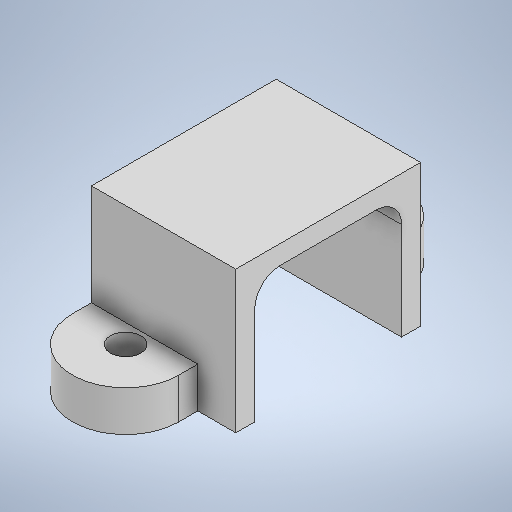
# Autodesk Inventor part: soporteMotor
Saved by Autodesk Inventor 2025.2 (Build 292293000, 293)
## iProperties
Created: 2025-06-11
Part Number: soporteMotor
Material: Generic
Document SubType Name: Modeling
Designer: cdavi
Density: 1 g/cm^3
Appearance: Default
Author: cdavi
Autodesk Inventor part; units mm, degrees
ref_plane "YZ Plane" through (0, 0, 0) normal (1, 0, 0) x (0, 1, 0)
ref_plane "XZ Plane" through (0, 0, 0) normal (0, 1, 0) x (-1, 0, 0)
ref_plane "XY Plane" through (0, 0, 0) normal (0, 0, 1) x (1, 0, 0)
sketch "Sketch1" plane through (0, 0, 0) normal (1, 0, 0) x (0, 1, 0)
  line L0 (11.2, 0) -> (11.2, -7.3)
  line L1 (11.2, -7.3) -> (0, -7.3)
  line L2 (9.7, 0) -> (9.7, -3.8)
  line L3 (7.7, -5.8) -> (0, -5.8)
  arc A0 (7.7, -5.8) -> (9.7, -3.8) centre (7.7, -3.8) ccw
  line L4 (0, -5.8) -> (0, -7.3)
  line L5 (0, 0) -> (11.2, 0) construction
  line L6 (11.2, 0) -> (11.2, 7.3)
  line L7 (11.2, 7.3) -> (0, 7.3)
  line L8 (9.7, 0) -> (9.7, 3.8)
  line L9 (7.7, 5.8) -> (0, 5.8)
  arc A1 (9.7, 3.8) -> (7.7, 5.8) centre (7.7, 3.8) ccw
  line L10 (0, 5.8) -> (0, 7.3)
  dimension "d2" = 5.8
  dimension "d4" = 1.5
  dimension "d5" = 2
  dimension "d6" = 11.2
  dimension "d7" = 1.5
  constraints: 22 end point, 6 symmetric about line, 4 point on circle, 3 vertical, 2 centre point, 2 horizontal alignment, 2 perpendicular, 2 tangent, 1 vertical alignment, 1 other
  measures "d2" distance from line of L5.start L3
  measures "d4" distance between parallel lines of L1 L3
  measures "d5" radius of A0
  measures "d6" distance from line of L5.start L0
  measures "d7" distance between parallel lines of L0 L2
extrude "Extrusion1" add sketch "Sketch1" along normal blind 11.4
sketch "Sketch3" plane through (0, 0, 0) normal (0, 1, 0) x (-1, 0, 0)
  line L0 (0, -7.3) -> (0, 7.3) projected
  line L1 (0, -7.3) -> (0, -8.8)
  line L2 (-8.4, -8.8) -> (-8.4, -7.3)
  line L3 (0, -7.3) -> (-11.4, -7.3) projected
  line L4 (0, -8.8) -> (-8.4, -8.8) construction
  arc A0 (-8.4, -8.8) -> (0, -8.8) centre (-4.2, -8.8) ccw
  circle A1 centre (-4.2, -8.8) radius 1.2
  point P0 (0, 0)
  dimension "d12" = 1.5
  dimension "d13" = 4.2
  dimension "d16" = 2.4
  constraints: 6 end point, 2 centre point, 2 point on circle, 2 vertical, 1 coincident, 1 horizontal, 1 point on line, 1 tangent
  measures "d12" distance from line of L3 L1.end
  measures "d13" radius of A0
  measures "d16" diameter of A1
extrude "Extrusion2" add sketch "Sketch3" along normal blind 3.2
mirror "Mirror1" about plane through (0, 0, 0) normal (0, 0, 1) of "Extrusion2"
body "Solid1"
